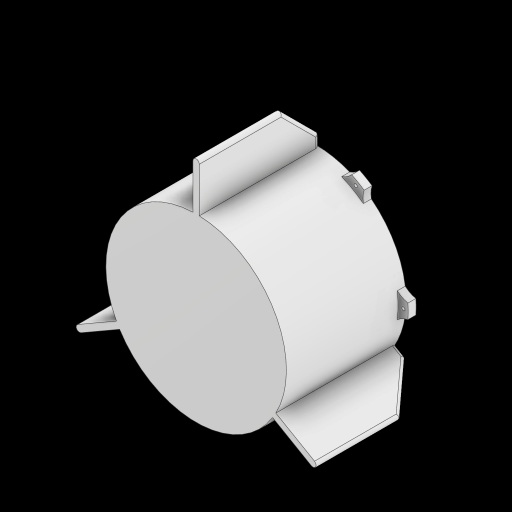
# Autodesk Inventor part: BackCapV2
Saved by Autodesk Inventor 2024 (Build 280153000, 153)
## iProperties
Created: 2026-04-12
Part Number: BackCapV2
Material: PVC-Piping
Document SubType Name: Modeling
Designer: Tanner
Density: 1.4 g/cm^3
Appearance: Smooth - White
Author: Tanner
## iProperties of the stored document BackCapV2_3DPrint.ipt
Created: 2026-04-13
Part Number: BackCapV2_3DPrint
Material: Generic
Document SubType Name: Modeling
Designer: Tanner
Density: 1 g/cm^3
Appearance: Default
Author: Tanner
Autodesk Inventor part; units mm, degrees
ref_plane "YZ Plane" through (0, 0, 0) normal (1, 0, 0) x (0, 1, 0)
ref_plane "XZ Plane" through (0, 0, 0) normal (0, 1, 0) x (-1, 0, 0)
ref_plane "XY Plane" through (0, 0, 0) normal (0, 0, 1) x (1, 0, 0)
sketch "Sketch1" plane through (0, 0, 0) normal (1, 0, 0) x (0, 1, 0)
  line L0 (-107.6, 0) -> (107.6, 0) construction
  line L1 (105.4894, -30) -> (101.5516, -30) construction
  line L2 (108.1, 1.5) -> (108.1, -29)
  line L3 (108.1, -29) -> (113.1, -29)
  line L4 (113.1, -29) -> (113.1, 121)
  line L5 (98.1, 1.5) -> (98.1, 7.5)
  line L6 (113.1, 121) -> (0, 121)
  line L7 (108.1, 17.5) -> (108.1, 116)
  line L8 (98.1, 7.5) -> (108.1, 17.5)
  line L9 (98.1, 7.5) -> (112.2421, 7.5) construction
  line L10 (108.1, 116) -> (0, 116)
  line L11 (0, 116) -> (0, 121)
  line L12 (107.6, 1.5) -> (107.6, -254) construction
  line L13 (99.6, -254) -> (99.6, 1.5) construction
  line L14 (107.6, 1.5) -> (-107.6, 1.5) construction
  line L15 (108.1, 1.5) -> (98.1, 1.5)
  point P0 (0, 0)
  point P1 (101.6, 0)
  point P2 (0, 118.5)
  point P3 (0, 0)
  dimension "d1" = 5
  dimension "d3" = 1
  dimension "d4" = 10
  dimension "d5" = 150
  dimension "d7" = 45
  dimension "d8" = 5
  dimension "d10" = 0.5
  dimension "d11" = 6
  constraints: 26 end point, 6 vertical, 3 horizontal, 2 collinear, 2 midpoint, 2 perpendicular, 1 equal length, 1 horizontal alignment, 1 point on line, 1 vertical alignment, 5 other
  measures "d1" distance between parallel lines of L2 L4
  measures "d3" distance between parallel lines of L1 L3
  measures "d4" distance of L2.start L5.start
  measures "d5" distance of L3.end L4.end
  measures "d7" angle of L9 L8
  measures "d8" distance between parallel lines of L6 L10
  measures "d10" distance between parallel lines of L12 L2
  measures "d11" distance of L5.start L5.end
revolve "Revolution1" add sketch "Sketch1" angle 360 about axis through (0, 0, 116) along (0, 0, 1)
sketch "Sketch3" plane through (0, 0, -29) normal (0, 0, -1) x (-1, 0, 0)
  circle A0 centre (-119.75, 0) radius 2.665 construction
  arc A1 (-103.5653, 29.1889) -> (-103.5653, -29.1889) centre (0, 0) ccw construction
  arc A2 (-103.5653, -29.1889) -> (-125.2771, -9) centre (-130.9966, -36.9202) ccw projected
  arc A3 (-125.2771, 9) -> (-125.2771, -9) centre (0, 0) ccw projected
  arc A4 (-125.2771, 9) -> (-103.5653, 29.1889) centre (-130.9966, 36.9202) ccw projected
  circle A5 centre (0, 0) radius 113.1 projected
  circle A6 centre (0, 0) radius 108.1 construction
  circle A7 centre (-119.75, 0) radius 2.125
  point P0 (0, 0)
  point P1 (-125.2771, 9)
  point P2 (-125.2771, -9)
  point P3 (-112.0098, -15.6658)
  point P4 (-112.0098, 15.6658)
  dimension "d12" = 4.25
  constraints: 1 centre point, 1 coincident
  measures "d12" diameter of A7
extrude "Extrusion1" add sketch "Sketch3" against normal blind 10 contours A2 A3 A4 A5
pattern_circular "Circular Pattern1" count 6 over 360 about axis through (0, 0, 46) along (0, 0, 1) of "Extrusion1"
sketch "Sketch4" plane through (0, 0, -29) normal (0, 0, -1) x (-1, 0, 0)
  arc A0 (42.4379, 104.8362) -> (-42.4379, 104.8362) centre (0, 0) ccw construction
  circle A1 centre (0, 0) radius 108.1 construction
  arc A2 (4, 113.0292) -> (-4, 113.0292) centre (0, 0) ccw
  line L0 (-4, 113.0292) -> (4, 113.0292) construction
  line L1 (4, 113.0292) -> (4, 173.0292)
  line L2 (-4, 113.0292) -> (-4, 173.0292)
  line L3 (-4, 173.0292) -> (4, 173.0292)
  point P0 (0, 0)
  point P1 (0, 113.0292)
  dimension "d19" = 8
  dimension "d20" = 60
  constraints: 8 end point, 2 concentric, 2 point on circle, 2 vertical, 1 centre point, 1 horizontal, 1 horizontal alignment, 1 midpoint, 1 perpendicular, 1 vertical alignment
  measures "d19" distance of L0.start L0.end
  measures "d20" distance of L0.end L1.end
extrude "Extrusion2" add sketch "Sketch4" against normal up to surface (150 mm away)
sketch "Sketch5" plane through (-4, 113.0292, -29) normal (-1, 0, 0) x (0, 0, 1)
  line L0 (0, 0) -> (0, 60) construction
  line L1 (150, 0) -> (0, 0) construction
  line L2 (0, 60) -> (150, 60) construction
  line L3 (0, 14) -> (46, 60)
  line L4 (0, 60) -> (150, 60) projected
  line L5 (0, 14) -> (0, 60)
  line L6 (0, 60) -> (46, 60)
  line L7 (150, 0) -> (150, 60) projected
  point P0 (29, -113.0292)
  point P1 (120, 75)
  dimension "d23" = 45
  dimension "d24" = 14
  constraints: 6 end point, 2 collinear, 1 point on line, 2 other
  measures "d23" angle of L0 L3
  measures "d24" distance from line of L3.start L1
extrude "Extrusion3" cut sketch "Sketch5" against normal through all
fillet "Fillet2" radius 4 6 edges at (-4, 120.0292, -29) (4, 120.0292, -29) (4, 150.0292, -6) (-4, 150.0292, -6) (4, 173.0292, 69) (-4, 173.0292, 69)
pattern_circular "Circular Pattern2" count 3 over 360 about axis through (0, 0, 46) along (0, 0, 1) of "Extrusion2", "Extrusion3", "Fillet2"
body "Solid1"
